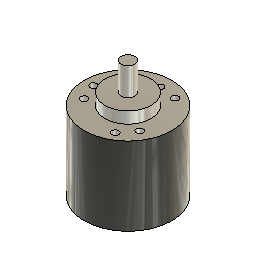
Encoder (Autodesk Fusion 360 design; units mm, degrees)
Autodesk Fusion 360 part; units mm, degrees
sketch "Skizze1" plane through (0, 0, 0) normal (0, 0, 1) x (1, 0, 0)
  circle A0 centre (0, 0) radius 19
  circle A1 centre (0, 0) radius 10
  circle A2 centre (0, 0) radius 3
  dimension "d1" = 38
  dimension "d2" = 20
  dimension "d3" = 6
  constraint coincident A0.centre A1.centre
  constraint concentric A0 A1
  measures "d1" diameter of A0
  measures "d2" diameter of A1
  measures "d3" diameter of A2
extrude "Extrusion3" add sketch "Skizze1" along normal blind 39 contours A2 makes body 1
extrude "Extrusion2" add sketch "Skizze1" along normal blind 39 separate body contours A1 makes body 2
extrude "Extrusion1" add sketch "Skizze1" along normal blind 34 separate body contours A0 makes body 3
extrude "Extrusion4" add 1 faces at (0.3505, -0.866, 39) along direction (0, 0, 1) blind 12 on bodies 1 bodies 1 3 2
sketch "Skizze2" plane through (0, 0, 34) normal (0, 0, 1) x (-1, 0, 0)
  circle A0 centre (0, 0) radius 10
  circle A1 centre (0, 0) radius 19
  line L0 (0, 0) -> (0, -14) construction
  line L1 (0, 0) -> (-7.5, -12.9904) construction
  line L2 (0, 0) -> (12.3693, 0) construction
  line L3 (0, 0) -> (15, 0) construction
  line L4 (0, 0) -> (12.1244, 7) construction
  line L5 (0, 0) -> (12.6491, 0) construction
  circle A2 centre (15, 0) radius 1.5
  circle A3 centre (12.1244, 7) radius 1.5
  circle A4 centre (0, -14) radius 1.5
  circle A5 centre (-7.5, -12.9904) radius 1.5
  line L6 (0, 0) -> (-12.1244, 7) construction
  line L7 (0, 0) -> (11.7072, 0) construction
  line L8 (0, 0) -> (-7.5, 12.9904) construction
  line L9 (0, 0) -> (13.6015, 0) construction
  circle A6 centre (-12.1244, 7) radius 1.5
  circle A7 centre (-7.5, 12.9904) radius 1.5
  dimension "d12" = 14
  dimension "d13" = 120
  dimension "d14" = 15
  dimension "d15" = 15
  dimension "d16" = 30
  dimension "d17" = 14
  dimension "d18" = 3
  dimension "d19" = 3
  dimension "d20" = 3
  dimension "d21" = 3
  dimension "d22" = 150
  dimension "d23" = 14
  dimension "d24" = 120
  dimension "d25" = 15
  dimension "d26" = 3
  dimension "d27" = 3
  constraint coincident A0.centre A1.centre
  constraint vertical L0
  constraint horizontal L2
  constraint perpendicular L0 L3
  constraint horizontal L5
  constraint coincident L3.end A2.centre
  constraint coincident L4.end A3.centre
  constraint coincident L0.end A4.centre
  constraint coincident L1.end A5.centre
  constraint horizontal L7
  constraint horizontal L9
  constraint coincident L6.end A6.centre
  constraint coincident L8.end A7.centre
  measures "d12" distance of A0.centre L0.end
  measures "d13" angle of L1 L2
  measures "d14" distance of A0.centre L1.end
  measures "d15" distance of A0.centre L3.end
  measures "d16" angle of L4 L5
  measures "d17" distance of A0.centre L4.end
  measures "d18" diameter of A2
  measures "d19" diameter of A3
  measures "d20" diameter of A4
  measures "d21" diameter of A5
  measures "d22" angle of L6 L7
  measures "d23" distance of A0.centre L6.end
  measures "d24" angle of L8 L9
  measures "d25" distance of A0.centre L8.end
  measures "d26" diameter of A6
  measures "d27" diameter of A7
extrude "Extrusion6" cut sketch "Skizze2" against normal blind 5 contours A5 bodies 3
extrude "Extrusion5" cut sketch "Skizze2" against normal blind 5 contours A4 bodies 3
extrude "Extrusion7" cut sketch "Skizze2" against normal blind 5 contours A6 bodies 3
extrude "Extrusion8" cut sketch "Skizze2" against normal blind 5 contours A7 bodies 3
extrude "Extrusion9" cut sketch "Skizze2" against normal blind 5 contours A3 bodies 3
extrude "Extrusion10" cut sketch "Skizze2" against normal blind 5 contours A2 bodies 3
